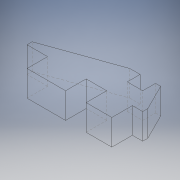
# Autodesk Inventor part: Support_carte_ground
Saved by Autodesk Inventor 2017 (Build 210142000, 142)
## iProperties
Part Number: Support_carte_ground
Material: Générique
Document SubType Name: Modeling
Designer: Darren
Density: 1 g/cm^3
Appearance: Par défaut
Author: Darren
Autodesk Inventor part; units mm, degrees
ref_plane "YZ Plane" through (0, 0, 0) normal (1, 0, 0) x (0, 1, 0)
ref_plane "XZ Plane" through (0, 0, 0) normal (0, 1, 0) x (-1, 0, 0)
ref_plane "XY Plane" through (0, 0, 0) normal (0, 0, 1) x (1, 0, 0)
sketch "Esquisse1" plane through (0, 0, 0) normal (0, 0, 1) x (1, 0, 0)
  line L0 (45, 0) -> (45, 2)
  line L1 (0, 2) -> (0, 0)
  line L2 (38, 12) -> (38, 7)
  line L3 (38, 7) -> (32, 7)
  line L4 (32, 7) -> (32, 12)
  line L5 (28, 12) -> (32, 12)
  line L6 (38, 12) -> (40, 12)
  line L7 (0, 2) -> (45, 2) construction
  line L8 (0, 2) -> (28, 12)
  line L9 (40, 12) -> (45, 2)
  line L10 (23, 0) -> (23, -8)
  line L11 (23, -8) -> (8, -8)
  line L12 (8, -8) -> (8, 0)
  line L13 (41, 0) -> (41, -8)
  line L14 (41, -8) -> (31, -8)
  line L15 (31, -8) -> (31, 0)
  line L16 (0, 0) -> (8, 0)
  line L17 (23, 0) -> (31, 0)
  line L18 (41, 0) -> (45, 0)
  dimension "d10" = 45
  dimension "d12" = 6
  dimension "d13" = 7
  dimension "d14" = 5
  dimension "d15" = 5
  dimension "d18" = 153.435
  dimension "d19" = 70.346
  dimension "d20" = 10
  dimension "d21" = 15
  dimension "d23" = 8
  dimension "d24" = 10
  dimension "d26" = 4
  dimension "d27" = 7
  dimension "d28" = 8
  dimension "d29" = 8
  dimension "d30" = 8
  dimension "d31" = 8
  constraints: 38 end point, 4 horizontal, 4 parallel, 3 perpendicular
  measures "d10" distance between parallel lines of L0 L1
  measures "d12" distance between parallel lines of L2 L4
  measures "d13" distance between parallel lines of L0 L2
  measures "d14" distance between parallel lines of L3 L6
  measures "d15" distance between parallel lines of L3 L5
  measures "d18" angle of L9 L0
  measures "d19" angle of L0 L8
  measures "d20" distance between parallel lines of L6 L7
  measures "d21" distance of L10.end L11.end
  measures "d23" distance between parallel lines of L1 L12
  measures "d24" distance of L13.end L14.end
  measures "d26" distance between parallel lines of L0 L13
  measures "d27" distance between parallel lines of L16 L3
  measures "d28" distance between parallel lines of L17 L11
  measures "d29" distance between parallel lines of L14 L17
  measures "d30" distance between parallel lines of L18 L14
  measures "d31" distance between parallel lines of L11 L16
extrude "Extrusion1" add sketch "Esquisse1" along normal blind 10
